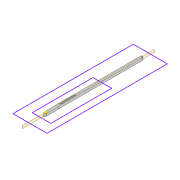
# Autodesk Inventor part: Part_8
Saved by Autodesk Inventor 2022 (Build 260153000, 153)
## iProperties
Created: 2022-04-26
Part Number: Part_8
Material: Generic
Document SubType Name: Modeling
Designer: dell
Density: 1 g/cm^3
Appearance: Default
Author: dell
Autodesk Inventor part; units mm, degrees
ref_plane "XZ Plane" through (0, 0, 0) normal (0, 1, 0) x (-1, 0, 0)
ref_plane "XY Plane" through (0, 0, 0) normal (0, 0, 1) x (1, 0, 0)
sketch "Sketch1" plane through (0, 0, 0) normal (0, 1, 0) x (-1, 0, 0)
  line L0 (0, 0) -> (0, -319.927) construction
  line L1 (-4, 0) -> (-4, -319.927)
  line L2 (4, -319.927) -> (4, 0)
  arc A0 (4, 0) -> (-4, 0) centre (0, 0) ccw
  arc A1 (-4, -319.927) -> (4, -319.927) centre (0, -319.927) ccw
  circle A2 centre (0, 0) radius 1.5
  circle A3 centre (0, -319.927) radius 1.5
  line L3 (0, -50.8) -> (0, -100) construction
  line L4 (-1.5, -50.8) -> (-1.5, -100)
  line L5 (1.5, -100) -> (1.5, -50.8)
  arc A4 (1.5, -50.8) -> (-1.5, -50.8) centre (0, -50.8) ccw
  arc A5 (-1.5, -100) -> (1.5, -100) centre (0, -100) ccw
  arc A6 (4, 0) -> (4, -40) centre (202.9975, -20) ccw
  arc A7 (-4, 0) -> (-4, -40) centre (194.9975, -20) ccw
  point P0 (0, -159.9635)
  point P1 (0, -75.4)
  dimension "d0" = 319.927
  dimension "d1" = 8
  dimension "d2" = 3
  dimension "d3" = 3
  dimension "d12" = 3
  dimension "d13" = 50.8
  dimension "d14" = 100
  dimension "d15" = 40
  dimension "d16" = 200
  dimension "d17" = 200
  constraints: 16 end point, 12 point on circle, 8 centre point, 8 tangent, 4 point on line, 2 coincident, 2 midpoint, 2 parallel, 1 horizontal alignment, 1 vertical
  measures "d0" distance of L0.start L0.end
  measures "d1" diameter of A1
  measures "d2" diameter of A2
  measures "d3" diameter of A3
  measures "d12" diameter of A5
  measures "d13" distance of A2.centre L3.start
  measures "d14" distance of L0.start L3.end
  measures "d15" vertical distance of A6.end L0.start
  measures "d16" radius of A6
  measures "d17" radius of A7
extrude "Extrusion1" add sketch "Sketch1" along normal blind 8 contours A0 A6 L2 A1 L1 | L1 A7
sketch "Sketch2" plane through (0, 0, 0) normal (0, -1, 0) x (1, 0, 0)
  arc A0 (4, -40) -> (4, 0) centre (-194.9975, -20) ccw projected
  arc A1 (4, 0) -> (-4, 0) centre (0, 0) ccw projected
  arc A2 (-4, -40) -> (-4, 0) centre (-202.9975, -20) ccw projected
  line L0 (-4, -319.927) -> (-4, -40) projected
  arc A3 (-4, -319.927) -> (4, -319.927) centre (0, -319.927) ccw projected
  line L1 (4, -40) -> (4, -319.927) projected
  circle A4 centre (0, 0) radius 1.5 projected
  circle A5 centre (0, -319.927) radius 1.5 projected
  arc A6 (1.5, -50.8) -> (-1.5, -50.8) centre (0, -50.8) ccw projected
  line L2 (1.5, -100) -> (1.5, -50.8) projected
  arc A7 (-1.5, -100) -> (1.5, -100) centre (0, -100) ccw projected
  line L3 (-1.5, -50.8) -> (-1.5, -100) projected
sketch "Sketch3" plane through (0, 8, 0) normal (0, 1, 0) x (1, 0, 0)
  line L0 (-21.634, 180.7321) -> (39.8396, 180.7321)
  line L1 (39.8396, 180.7321) -> (39.8396, -20.7362)
  line L2 (39.8396, -20.7362) -> (-21.634, -20.7362)
  line L3 (-21.634, -20.7362) -> (-21.634, 180.7321)
  line L4 (-50.5628, 342.9399) -> (62.0528, 342.9399)
  line L5 (62.0528, 342.9399) -> (62.0528, -55.3474)
  line L6 (62.0528, -55.3474) -> (-50.5628, -55.3474)
  line L7 (-50.5628, -55.3474) -> (-50.5628, 342.9399)
  point P0 (0, 0)
  constraints: 16 end point, 4 parallel, 2 horizontal, 2 perpendicular
body "Solid1"
